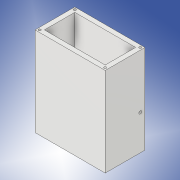
# Autodesk Inventor part: HA005
Saved by Autodesk Inventor 2017 SP1 (Build 210196100, 196)
## iProperties
Created: 2017-06-10
Part Number: HA005
Material: ABS Plastic
Document SubType Name: Modeling
Designer: Zach
Density: 1.06 g/cm^3
Appearance: CR White
Author: Zach
Autodesk Inventor part; units mm, degrees
ref_plane "YZ Plane" through (0, 0, 0) normal (1, 0, 0) x (0, 1, 0)
ref_plane "XZ Plane" through (0, 0, 0) normal (0, 1, 0) x (-1, 0, 0)
ref_plane "XY Plane" through (0, 0, 0) normal (0, 0, 1) x (1, 0, 0)
sketch "Sketch1" plane through (0, 0, 0) normal (0, 0, 1) x (1, 0, 0)
  line L0 (0, 0) -> (150, 0)
  line L1 (150, 0) -> (150, 200)
  line L2 (150, 200) -> (0, 200)
  line L3 (0, 200) -> (0, 0)
  dimension "d0" = 150
  dimension "d1" = 200
  constraints: 8 end point, 2 parallel, 1 horizontal, 1 perpendicular
  measures "d0" distance of L2.end L1.end
  measures "d1" distance of L1.end L0.end
extrude "Extrusion1" add sketch "Sketch1" along normal blind 20
sketch "Sketch2" plane through (150, 0, 0) normal (1, 0, 0) x (0, 0, -1)
  circle A0 centre (-10, 75) radius 3
  line L0 (0, 200) -> (-20, 200) projected
  point P0 (0, 0)
  point P1 (-10, 200)
  dimension "d4" = 6
  dimension "d5" = 75
  constraints: 1 centre point, 1 midpoint, 1 vertical alignment
  measures "d4" diameter of A0
  measures "d5" vertical distance of point (0, 0) A0.centre
extrude "Extrusion2" cut sketch "Sketch2" against normal through all
sketch "Sketch3" plane through (0, 0, 20) normal (0, 0, 1) x (1, 0, 0)
  line L0 (150, 0) -> (150, 200) projected
  line L1 (0, 200) -> (150, 200)
  line L2 (150, 200) -> (150, 0)
  line L3 (150, 0) -> (0, 0)
  line L4 (0, 0) -> (0, 200)
  point P0 (0, 0)
  constraints: 8 end point, 2 parallel, 1 coincident, 1 horizontal, 1 perpendicular
extrude "Extrusion3" add sketch "Sketch3" along normal blind 65
sketch "Sketch4" plane through (0, 0, 0) normal (0, -1, 0) x (1, 0, 0)
  circle A0 centre (37.5, 42.5) radius 12.5
  circle A1 centre (112.5, 42.5) radius 12.5
  line L0 (37.5, 42.5) -> (112.5, 42.5) construction
  line L1 (0, 0) -> (0, 85) projected
  line L2 (0, 85) -> (150, 85) projected
  point P0 (0, 42.5)
  point P1 (75, 42.5)
  point P2 (75, 85)
  dimension "d10" = 25
  dimension "d11" = 25
  dimension "d12" = 75
  constraints: 3 midpoint, 2 centre point, 2 end point, 1 horizontal, 1 horizontal alignment, 1 vertical alignment
  measures "d10" diameter of A0
  measures "d11" diameter of A1
  measures "d12" distance of L0.end L0.start
extrude "Extrusion4" cut sketch "Sketch4" against normal blind 100
sketch "Sketch5" plane through (0, 200, 0) normal (0, 1, 0) x (1, 0, 0)
  line L0 (150, 0) -> (0, 0) projected
  line L1 (0, 0) -> (0, -85) projected
  line L2 (150, -85) -> (0, -85) projected
  line L3 (150, 0) -> (150, -85) projected
  line L4 (140, -75) -> (10, -75)
  line L5 (10, -75) -> (10, -10)
  line L6 (10, -10) -> (140, -10)
  line L7 (140, -10) -> (140, -75)
  point P0 (0, 0)
  dimension "d15" = 10
  constraints: 8 end point, 3 other
  measures "d15" distance between parallel lines of L3 L7
extrude "Extrusion5" cut sketch "Sketch5" against normal blind 190 contours L4 L5 L6 L7
sketch "Sketch6" plane through (0, 0, 0) normal (-1, 0, 0) x (0, 0, 1)
  line L0 (0, 200) -> (85, 200) projected
  line L1 (0, 200) -> (0, 0) projected
  line L2 (85, 200) -> (0, 200)
  line L3 (0, 200) -> (0, 190)
  line L4 (0, 190) -> (85, 190)
  line L5 (85, 190) -> (85, 200)
  dimension "d18" = 10
  constraints: 8 end point, 2 parallel, 1 horizontal, 1 perpendicular, 1 point on line
  measures "d18" distance of L3.end L2.end
extrude "Extrusion6" cut sketch "Sketch6" against normal through all
sketch "Sketch7" plane through (0, 190, 85) normal (0, 1, 0) x (1, 0, 0)
  line L0 (150, 85) -> (150, 0) construction
  line L1 (0, 85) -> (150, 85) construction
  line L2 (0, 0) -> (0, 85) construction
  line L3 (150, 0) -> (0, 0) construction
  line L4 (140, 10) -> (140, 75) construction
  line L5 (10, 10) -> (140, 10) construction
  line L6 (10, 75) -> (10, 10) construction
  line L7 (140, 75) -> (10, 75) construction
  line L8 (145, 5) -> (145, 80) construction
  line L9 (145, 80) -> (5, 80) construction
  line L10 (5, 80) -> (5, 5) construction
  line L11 (5, 5) -> (145, 5) construction
  circle A0 centre (145, 5) radius 2.5
  circle A1 centre (145, 80) radius 2.5
  circle A2 centre (5, 80) radius 2.5
  circle A3 centre (5, 5) radius 2.5
  point P0 (0, 85)
  dimension "d21" = 5
  dimension "d22" = 5
  dimension "d23" = 5
  dimension "d24" = 5
  dimension "d25" = 5
  constraints: 8 end point, 4 centre point, 4 coincident, 3 other
  measures "d21" distance between parallel lines of L0 L8
  measures "d22" diameter of A0
  measures "d23" diameter of A1
  measures "d24" diameter of A2
  measures "d25" diameter of A3
extrude "Extrusion7" cut sketch "Sketch7" against normal blind 25
body "Solid1"
